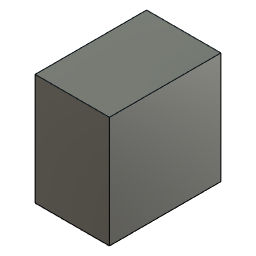
bureau v1 (Autodesk Fusion 360 design; units mm, degrees)
Autodesk Fusion 360 part; units mm, degrees
sketch "Esquisse1" plane through (0, 0, 0) normal (0, 1, 0) x (1, 0, 0)
  line L0 (-400, 400) -> (400, 400)
  line L1 (400, 400) -> (400, -400)
  line L2 (400, -400) -> (-400, -400)
  line L3 (-400, -400) -> (-400, 400)
  line L4 (-400, 400) -> (400, -400) construction
  line L5 (400, 400) -> (-400, -400) construction
  dimension "d1" = 800
  dimension "d2" = 800
  constraint horizontal L0
  constraint perpendicular L0 L1
  constraint parallel L0 L2
  constraint parallel L1 L3
  constraint coincident L4 origin
  constraint coincident L5 origin
  measures "d1" distance of L0.start L0.end
  measures "d2" distance of L0.end L1.end
extrude "Extrusion1" add sketch "Esquisse1" along normal blind 1200
extrude "Extrusion2" add 1 faces at (133.3333, 400, 400) along direction (0, 0, 1) blind 200
extrude "Extrusion3" add 1 faces at (133.3333, 400, 600) along direction (0, 0, 1) blind 200
sketch "Esquisse2" plane through (0, 1200, 0) normal (0, 1, 0) x (-1, 0, 0)
  line L0 (-400, 800) -> (-400, -400)
  line L1 (-400, -400) -> (400, -400)
  line L2 (400, -400) -> (400, 800)
  line L3 (400, 800) -> (-400, 800)
